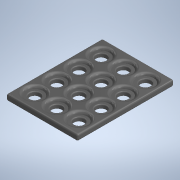
# Autodesk Inventor part: Test1
Saved by Autodesk Inventor 2020 (Build 240168000, 168)
## iProperties
Part Number: Test1
Material: Типовой
Document SubType Name: Обычные детали
Designer: User
Appearance: По умолчанию
Author: User
Autodesk Inventor part; units mm, degrees
ref_plane "Плоскость YZ" through (0, 0, 0) normal (1, 0, 0) x (0, 1, 0)
ref_plane "Плоскость XZ" through (0, 0, 0) normal (0, 1, 0) x (-1, 0, 0)
ref_plane "Плоскость XY" through (0, 0, 0) normal (0, 0, 1) x (1, 0, 0)
sketch "Эскиз1" plane through (0, 0, 0) normal (0, 1, 0) x (-1, 0, 0)
  line L0 (9.1667, 12.5) -> (-9.1667, 12.5)
  line L1 (-9.1667, 12.5) -> (-9.1667, -12.5)
  line L2 (-9.1667, -12.5) -> (9.1667, -12.5)
  line L3 (9.1667, -12.5) -> (9.1667, 12.5)
  line L4 (9.1667, 12.5) -> (-9.1667, -12.5) construction
  line L5 (-9.1667, 12.5) -> (9.1667, -12.5) construction
  line L6 (10.7667, 14.5) -> (-10.7667, 14.5)
  line L7 (-10.7667, 14.5) -> (-10.7667, -14.5)
  line L8 (-10.7667, -14.5) -> (10.7667, -14.5)
  line L9 (10.7667, -14.5) -> (10.7667, 14.5)
  line L10 (10.7667, 14.5) -> (-10.7667, -14.5) construction
  line L11 (-10.7667, 14.5) -> (10.7667, -14.5) construction
  circle A0 centre (6.6667, 10) radius 1.5
  circle A1 centre (6.6667, 3.3333) radius 1.5
  circle A2 centre (6.6667, -3.3333) radius 1.5
  circle A3 centre (6.6667, -10) radius 1.5
  circle A4 centre (0, 10) radius 1.5
  circle A5 centre (0, 3.3333) radius 1.5
  circle A6 centre (0, -3.3333) radius 1.5
  circle A7 centre (0, -10) radius 1.5
  circle A8 centre (-6.6667, 10) radius 1.5
  circle A9 centre (-6.6667, 3.3333) radius 1.5
  circle A10 centre (-6.6667, -3.3333) radius 1.5
  circle A11 centre (-6.6667, -10) radius 1.5
  point P0 (0, 0)
  dimension "d0" = 18.3333
  dimension "d1" = 25
  dimension "d2" = 1.6
  dimension "d3" = 2
  dimension "d4" = 3
  dimension "d5" = 2.5
  dimension "d6" = 2.5
  dimension "d9" = 6.6667
  dimension "d12" = 6.6667
  constraints: 24 end point, 12 centre point, 4 midpoint, 4 parallel, 3 horizontal, 2 perpendicular, 1 vertical, 22 other
  measures "d0" distance of L2.end L1.end
  measures "d1" distance of L1.end L0.end
  measures "d2" distance between parallel lines of L3 L9
  measures "d3" distance between parallel lines of L2 L8
  measures "d4" diameter of A0
  measures "d5" distance from line of A0.centre L3
  measures "d6" distance from line of L0 A0.centre
  measures "d9" distance of A0.centre A1.centre
  measures "d12" distance of A0.centre A4.centre
extrude "Выдавливание1" add sketch "Эскиз1" along normal blind 1.8 contours L3 L2 L1 L0 | L9 L8 L7 L6
fillet "Сопряжение1" radius 0.5 12 edges at (0, 1.8, 14.5) (10.7667, 1.8, 0) (10.7667, 0, 0) (0, 0, 14.5) (10.7667, 0.9, 14.5) (0, 1.8, -14.5) (0, 0, -14.5) (10.7667, 0.9, -14.5) (-10.7667, 0.9, -14.5) (-10.7667, 1.8, 0) (-10.7667, 0, 0) (-10.7667, 0.9, 14.5)
sketch "Эскиз2" plane through (0, 1.8, 0) normal (0, 1, 0) x (1, 0, 0)
  circle A0 centre (6.6667, 10) radius 1.5 projected
  circle A1 centre (6.6667, -3.3333) radius 1.5 projected
  circle A2 centre (0, 10) radius 1.5 projected
  circle A3 centre (0, 3.3333) radius 1.5 projected
  circle A4 centre (0, -3.3333) radius 1.5 projected
  circle A5 centre (0, -10) radius 1.5 projected
  circle A6 centre (-6.6667, 10) radius 1.5 projected
  circle A7 centre (-6.6667, 3.3333) radius 1.5 projected
  circle A8 centre (-6.6667, -3.3333) radius 1.5 projected
  circle A9 centre (-6.6667, -10) radius 1.5 projected
  circle A10 centre (6.6667, -10) radius 1.5 projected
  circle A11 centre (6.6667, 3.3333) radius 1.5 projected
  line L0 (10.2667, 14) -> (10.2667, -14) projected
  line L1 (-10.2667, 14) -> (10.2667, 14) projected
  line L2 (-10.2667, -14) -> (-10.2667, 14) projected
  line L3 (10.2667, -14) -> (-10.2667, -14) projected
  circle A12 centre (6.6667, 10) radius 1.5 projected
  circle A13 centre (6.6667, 10) radius 2.5
  point P0 (0, 0)
  dimension "d18" = 1
  constraints: 1 centre point, 1 coincident
  measures "d18" radial gap between concentric circles of A0 A13
extrude "Выдавливание2" cut sketch "Эскиз2" against normal blind 0.7 contours A13
fillet "Сопряжение2" radius 1 1 edges at (4.1667, 1.8, -10)
pattern_linear "Прямоуг.массив1" count 4 spacing 6.6667 along (0, 0, 1) count 3 spacing 6.6667 along (-1, 0, 0) of "Выдавливание2", "Сопряжение2"
fillet "Сопряжение3" radius 0.3 12 edges at (-5.1667, 1.1, 10) (-5.1667, 1.1, 3.3333) (-5.1667, 1.1, -3.3333) (-5.1667, 1.1, -10) (1.5, 1.1, -10) (8.1667, 1.1, -10) (8.1667, 1.1, -3.3333) (1.5, 1.1, -3.3333) (1.5, 1.1, 3.3333) (1.5, 1.1, 10) (8.1667, 1.1, 10) (8.1667, 1.1, 3.3333)
equation "\"d6\" = d5"
